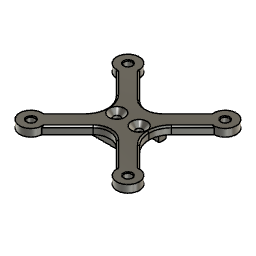
load_cell_contraption (Autodesk Fusion 360 archive; units mm, degrees)
design "Canon Weight Adapter"
Autodesk Fusion 360 part; units mm, degrees
sketch "Skizze1" plane through (0, 0, 0) normal (0, 0, 1) x (1, 0, 0)
  circle A0 centre (0, 0) radius 2.25
  line L0 (0, 0) -> (15, 0) construction
  circle A1 centre (15, 0) radius 2.25
  line L1 (-6.5, 6.5) -> (21.5, 6.5)
  line L2 (21.5, 0.0034) -> (21.5, -0.0034)
  line L3 (21.5, -6.5) -> (-6.5, -6.5)
  line L4 (-6.5, -0.0034) -> (-6.5, 0.0034)
  line L5 (21.5, -11.5) -> (-6.5, -11.5)
  line L6 (-6.5, 11.5) -> (21.5, 11.5)
  line L7 (-6.5, 6.5) -> (-6.5, 11.5)
  line L8 (-6.5, -6.5) -> (-6.5, -11.5)
  line L9 (21.5, 6.5) -> (21.5, 11.5)
  line L10 (21.5, -6.5) -> (21.5, -11.5)
  circle A2 centre (-25.006, 32.4943) radius 7.5
  circle A3 centre (-25.006, 32.4943) radius 2.5
  line L11 (-25.006, 32.4943) -> (7.5, 0) construction
  circle A4 centre (7.5, 0) radius 5.5 construction
  circle A5 centre (-25.006, 32.4943) radius 5.5 construction
  line L12 (-21.1176, 36.3841) -> (-0.2768, 15.5508)
  line L13 (-28.8944, 28.6045) -> (-10.8953, 10.6119)
  line L14 (-6.5, 0) -> (21.5, 0) construction
  line L15 (7.5, 11.5) -> (7.5, -11.5) construction
  circle A6 centre (40.006, 32.4943) radius 7.5
  circle A7 centre (40.006, 32.4943) radius 2.5
  line L16 (36.1176, 36.3841) -> (15.2768, 15.5508)
  line L17 (43.8944, 28.6045) -> (25.8953, 10.6119)
  circle A8 centre (40.006, -32.4943) radius 7.5
  line L18 (36.1176, -36.3841) -> (15.2768, -15.5508)
  line L19 (43.8944, -28.6045) -> (25.8953, -10.6119)
  circle A9 centre (40.006, -32.4943) radius 2.5
  line L20 (-21.1176, -36.3841) -> (-0.2768, -15.5508)
  line L21 (-28.8944, -28.6045) -> (-10.8953, -10.6119)
  circle A10 centre (-25.006, -32.4943) radius 7.5
  circle A11 centre (-25.006, -32.4943) radius 2.5
  arc A12 (-6.5, 0.0034) -> (-10.8953, 10.6119) centre (-21.5, 0.0034) ccw
  arc A13 (-10.8953, -10.6119) -> (-6.5, -0.0034) centre (-21.5, -0.0034) ccw
  arc A14 (25.8953, 10.6119) -> (21.5, 0.0034) centre (36.5, 0.0034) ccw
  arc A15 (21.5, -0.0034) -> (25.8953, -10.6119) centre (36.5, -0.0034) ccw
  arc A16 (-0.2768, 15.5508) -> (15.2768, 15.5508) centre (7.5, 23.3303) ccw
  arc A17 (15.2768, -15.5508) -> (-0.2768, -15.5508) centre (7.5, -23.3303) ccw
  dimension "d1" = 4.5
  dimension "d2" = 15
  dimension "d3" = 4.5
  dimension "d4" = 28
  dimension "d5" = 6.5
  dimension "d6" = 6.5
  dimension "d15" = 7.5
  dimension "d16" = 5
  dimension "d17" = 11
  dimension "d18" = 11
  dimension "d19" = 15
  dimension "d20" = 15
  dimension "d21" = 15
  dimension "d22" = 15
  dimension "d23" = 11
  dimension "d24" = 11
  constraint coincident A0.centre L0.start
  constraint horizontal L0
  constraint coincident L0.end A1.centre
  constraint horizontal L1
  constraint vertical L2
  constraint horizontal L3
  constraint vertical L4
  constraint perpendicular L6 L7
  constraint perpendicular L5 L8
  constraint perpendicular L6 L9
  constraint perpendicular L5 L10
  constraint concentric A2 A3
  constraint coincident A2.centre A3.centre
  constraint midpoint L0 L11.end
  constraint coincident L11.end A4.centre
  constraint concentric A3 A5
  constraint coincident A5 L12.start
  constraint tangent A4 L12
  constraint tangent A5 L12
  constraint coincident A5 L13.start
  constraint tangent A4 L13
  constraint tangent A5 L13
  constraint midpoint L6 L15.start
  constraint midpoint L5 L15.end
  constraint symmetric A2 L15 A6
  constraint symmetric A3 L15 A7
  constraint symmetric L12.start L15 L16.start
  constraint symmetric L13.start L15 L17.start
  constraint symmetric L0 A2 A10
  constraint symmetric L0 A3 A11
  constraint symmetric L0 L12.start L20.start
  constraint symmetric L0 L13.start L21.start
  constraint symmetric L0 A6 A8
  constraint symmetric L0 A7 A9
  constraint symmetric L0 L16.start L18.start
  constraint symmetric L0 L17.start L19.start
  constraint coincident L4 L14.start
  constraint coincident L1.start L4
  constraint tangent L13 A12
  constraint tangent L4 A12
  constraint coincident L3.end L4
  constraint tangent L21 A13
  constraint tangent L4 A13
  constraint coincident L2 L14.end
  constraint coincident L1.end L2
  constraint tangent L17 A14
  constraint tangent L2 A14
  constraint coincident L3.start L2
  constraint tangent L19 A15
  constraint tangent L2 A15
  constraint tangent L12 A16
  constraint tangent L16 A16
  constraint tangent L20 A17
  constraint tangent L18 A17
  measures "d1" diameter of A0
  measures "d2" distance of A0.centre L0.end
  measures "d3" diameter of A1
  measures "d4" distance of L1.start L1.end
  measures "d5" distance of A0.centre L1
  measures "d6" distance of A0.centre L4
  measures "d15" radius of A2
  measures "d16" diameter of A3
  measures "d17" diameter of A4
  measures "d18" diameter of A5
  measures "d19" radius of A12
  measures "d20" radius of A13
  measures "d21" radius of A14
  measures "d22" radius of A15
  measures "d23" radius of A16
  measures "d24" radius of A17
extrude "Extrusion1" add sketch "Skizze1" against normal blind 5 contours L1 L6 L7 L9 | L3 L5 L8 L10 makes body 1 at (12.1667, 9.8333, 0) makes body 2 at (12.1667, -11.5, -1.6667)
extrude "Extrusion2" add sketch "Skizze1" along normal blind 5 contours L1 L6 L7 L9 | L2 L4 A2 L12 L13 A6 L16 L17 A8 L18 L19 L20 L21 A10 A12 A13 A14 A15 A16 A17 | L3 L5 L8 L10 bodies 1 2
chamfer "Fase1" distance 3 angle 45 2 edges at (-2.0977, 0.8136, 5) (12.9023, 0.8136, 5) on bodies 1
extrude "Extrusion3" add sketch "Skizze1" along normal blind 5 contours A6 | A8 | A2 | A10 bodies 1
chamfer "Fase2" distance 1 angle 45 20 edges at (23.8941, 24.165, 5) (7.5, 12.3303, 5) (-8.8941, 24.165, 5) (33.0917, 17.8058, 5) (33.0917, -17.8058, 5) (22.6423, -5.7449, 5) (21.5, 0, 5) (22.6423, 5.7449, 5) (45.3103, 37.7967, 5) (23.8941, -24.165, 5) (-8.8941, -24.165, 5) (7.5, -12.3303, 5) (45.3103, -37.7967, 5) (-30.3103, -37.7967, 5) (-18.0917, -17.8058, 5) (-18.0917, 17.8058, 5) (-7.6423, 5.7449, 5) (-6.5, 0, 5) (-7.6423, -5.7449, 5) (-30.3103, 37.7967, 5) on bodies 1
extrude "Extrusion4" add sketch "Skizze1" along normal blind 5 contours A6 | A8 | A2 | A10 bodies 1
chamfer "Fase3" distance 0.5 angle 45 4 edges at (37.6752, -31.5903, 5) (-27.3368, -31.5903, 5) (-27.3368, 33.3984, 5) (37.6752, 33.3984, 5) on bodies 1
chamfer "Fase4" distance 0.5 angle 45 4 edges at (7.5, 6.5, -5) (7.5, -6.5, -5) (7.5, -11.5, -5) (7.5, 11.5, -5) on bodies 1
equation "d4 = 15 mm + 13 mm"

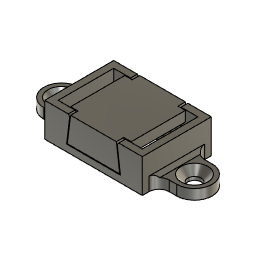
design "HX711 Cover"
Autodesk Fusion 360 part; units mm, degrees
sketch "Skizze1" plane through (0, 0, 0) normal (0, 0, 1) x (1, 0, 0)
  line L0 (0, 0) -> (25, 0)
  line L1 (25, 0) -> (25, 16.5)
  line L2 (25, 16.5) -> (0, 16.5)
  line L3 (0, 16.5) -> (0, 0)
  line L4 (3.5, 16.5) -> (3.5, 0)
  line L5 (21.5, 16.5) -> (21.5, 0)
  line L6 (-2, -2) -> (27, -2)
  line L7 (27, -2) -> (27, 18.5)
  line L8 (27, 18.5) -> (-2, 18.5)
  line L9 (-2, 18.5) -> (-2, -2)
  line L10 (5.5, 18.5) -> (5.5, -2)
  line L11 (19.5, 18.5) -> (19.5, -2)
  line L12 (12.5, -2) -> (12.5, 18.5) construction
  line L13 (12.5, 8.25) -> (27, 8.25) construction
  line L14 (27, 8.25) -> (32.25, 8.25) construction
  circle A0 centre (32.25, 8.25) radius 5.25
  circle A1 centre (32.25, 8.25) radius 3.25
  line L15 (32.25, 3) -> (27, 3)
  line L16 (32.25, 13.5) -> (27, 13.5)
  line L17 (-2, 8.25) -> (-7.25, 8.25) construction
  circle A2 centre (-7.25, 8.25) radius 3.25
  circle A3 centre (-7.25, 8.25) radius 5.25
  line L18 (-7.25, 3) -> (-2, 3)
  line L19 (-7.25, 13.5) -> (-2, 13.5)
  circle A4 centre (32.25, 8.25) radius 2
  circle A5 centre (-7.25, 8.25) radius 2
  line L20 (23, 14.5) -> (2, 14.5)
  line L21 (2, 14.5) -> (2, 2)
  line L22 (2, 2) -> (23, 2)
  line L23 (23, 2) -> (23, 14.5)
  dimension "d1" = 25
  dimension "d2" = 16.5
  dimension "d3" = 3.5
  dimension "d4" = 3.5
  dimension "d5" = 2
  dimension "d8" = 2
  dimension "d9" = 2
  dimension "d36" = 5.25
  dimension "d37" = 6.5
  dimension "d38" = 4
  dimension "d39" = 4
  dimension "d48" = -2
  constraint horizontal L0
  constraint vertical L1
  constraint horizontal L2
  constraint vertical L3
  constraint coincident L0.start L3.end
  constraint coincident L2 L4.start
  constraint coincident L0 L4.end
  constraint perpendicular L0 L4
  constraint coincident L2 L5.start
  constraint coincident L0 L5.end
  constraint perpendicular L0 L5
  constraint coincident L8 L10.start
  constraint coincident L6 L10.end
  constraint perpendicular L6 L10
  constraint coincident L8 L11.start
  constraint coincident L6 L11.end
  constraint perpendicular L6 L11
  constraint midpoint L6 L12.start
  constraint midpoint L8 L12.end
  constraint midpoint L12 L13.start
  constraint midpoint L7 L13.end
  constraint perpendicular L7 L14
  constraint coincident L14.end A0.centre
  constraint coincident L13.end A0
  constraint coincident A0 L15.start
  constraint coincident L7 L15.end
  constraint tangent A0 L15
  constraint perpendicular L7 L15
  constraint coincident A0 L16.start
  constraint coincident L7 L16.end
  constraint tangent A0 L16
  constraint perpendicular L7 L16
  constraint symmetric L12 L13.end L17.start
  constraint symmetric L12 L14.end L17.end
  constraint symmetric L12 A0 A3
  constraint symmetric L12 A1 A2
  constraint symmetric L12 L15.start L18.start
  constraint symmetric L12 L15.end L18.end
  constraint symmetric L12 L16.start L19.start
  constraint symmetric L12 L16.end L19.end
  constraint concentric A1 A4
  constraint concentric A2 A5
  measures "d1" distance of L0.start L0.end
  measures "d2" distance of L0.start L2.end
  measures "d3" distance of L3 L4
  measures "d4" distance of L1 L5
  measures "d8" distance of L4 L10
  measures "d9" distance of L5 L11
  measures "d36" distance of L13.end L14.end
  measures "d37" diameter of A1
  measures "d38" diameter of A4
  measures "d39" diameter of A5
extrude "Extrusion1" add sketch "Skizze1" against normal blind 2 contours L0 L2 L3 L4 L20 L21 L22 | L0 L2 L3 L6 L8 L9 L10 | L0 L4 L10 L22 | L0 L10 L11 L22 | L0 L6 L10 L11 | L4 L20 L21 L22 | L4 L10 L20 L22 | L2 L4 L10 L20 | L0 L5 L11 L22 | L0 L1 L2 L6 L7 L8 L11 | L10 L11 L20 L22 | L2 L8 L10 L11 | L2 L10 L11 L20 | L0 L1 L2 L5 L20 L22 L23 | L5 L11 L20 L22 | L2 L5 L11 L20 | L5 L20 L22 L23 makes body 1
extrude "Extrusion2" add sketch "Skizze1" along normal blind 6 contours L0 L2 L3 L6 L8 L9 L10 | L0 L1 L2 L6 L7 L8 L11 bodies 1
move_body "Verschieben1" bodies 1 to x (1, 0, 0) y (0, 1, 0) z (0, 0, 1) at (0, 0, -6)
extrude "Extrusion3" add sketch "Skizze1" along normal blind 2 contours L0 L2 L3 L6 L8 L9 L10 | L0 L1 L2 L6 L7 L8 L11 bodies 1
move_body "Verschieben2" bodies 1 to x (1, 0, 0) y (0, 1, 0) z (0, 0, 1) at (0, 0, -2)
extrude "Extrusion4" add sketch "Skizze1" against normal blind 2 separate body contours L0 L4 L10 L22 | L0 L10 L11 L22 | L0 L6 L10 L11 | L4 L10 L20 L22 | L2 L4 L10 L20 | L0 L5 L11 L22 | L10 L11 L20 L22 | L2 L8 L10 L11 | L2 L10 L11 L20 | L5 L11 L20 L22 | L2 L5 L11 L20 makes body 2
extrude "Extrusion5" add sketch "Skizze1" against normal blind 8 contours L0 L6 L10 L11 | L2 L8 L10 L11 bodies 2
sketch "Skizze2" plane through (0, 18.5, 0) normal (0, 1, 0) x (-1, 0, 0)
  line L0 (-27, 0) -> (-27, -10)
  line L1 (-27, -10) -> (2, -10)
  line L2 (2, -10) -> (2, 0)
  line L3 (2, 0) -> (-5.5, 0)
  line L4 (-5.5, 0) -> (-5.5, -8)
  line L5 (-5.5, -8) -> (-19.5, -8)
  line L6 (-19.5, -8) -> (-19.5, 0)
  line L7 (-19.5, 0) -> (-27, 0)
  line L8 (-19.5, 0) -> (-20.5, -8)
  line L9 (-20.5, -8) -> (-19.5, -8)
  line L10 (-5.5, -8) -> (-4.5, -8)
  line L11 (-4.5, -8) -> (-5.5, 0)
  line L12 (-19.5, -8) -> (-5.5, -8)
  line L13 (-19.3015, -0.0248) -> (-20.2734, -7.8)
  line L14 (-20.2734, -7.8) -> (-19.5, -7.8)
  line L15 (-19.5, -7.8) -> (-5.5, -7.8)
  line L16 (-5.5, -7.8) -> (-4.7266, -7.8)
  line L17 (-4.7266, -7.8) -> (-5.6985, -0.0248)
  line L18 (-19.5, 0) -> (-5.5, 0)
  line L19 (-5.6985, -0.0248) -> (-5.7016, 0)
  line L20 (-19.3015, -0.0248) -> (-19.2984, 0)
  dimension "d18" = -0.2
  constraint coincident L6.end L7.start
  constraint coincident L5.end L6.start
  constraint coincident L4.end L5.start
  constraint perpendicular L4 L10
  constraint coincident L3.end L4.start
  constraint parallel L17 L19
  constraint parallel L13 L20
  constraint coincident L18 L20.end
  constraint coincident L18 L19.end
extrude "Extrusion6" cut sketch "Skizze2" against normal blind 25 contours L6 L8 L9 L13 L14 | L6 L13 L14 | L4 L10 L11 L16 L17 | L4 L16 L17 bodies 1
extrude "Extrusion7" cut sketch "Skizze2" against normal blind 34 contours L4 L5 L6 L12 L15 bodies 2
extrude "Extrusion8" add sketch "Skizze2" against normal blind 20.5 contours L6 L13 L14 | L4 L16 L17 bodies 2
extrude "Extrusion9" cut sketch "Skizze2" against normal blind 18.5 contours L6 L13 L14 | L4 L16 L17 bodies 2
extrude "Extrusion10" add sketch "Skizze2" against normal blind 2 separate body contours L6 L13 L14 | L4 L16 L17 makes body 3 at (4.9844, 17.8333, -5.7375) makes body 4 at (19.7578, 17.8333, -3.675)
extrude "Extrusion11" cut sketch "Skizze2" against normal blind 21.5 contours L6 L13 L18 L20 | L4 L17 L18 L19 bodies 2
extrude "Extrusion12" add sketch "Skizze2" against normal blind 18.5 separate body contours L6 L13 L18 L20 | L4 L17 L18 L19 makes body 5 at (19.4328, 12.3333, -1.075) makes body 6 at (5.5672, 12.3333, -1.075)
extrude "Extrusion13" cut sketch "Skizze2" against normal blind 2 contours L6 L13 L18 L20 | L4 L17 L18 L19 bodies 5 6
combine "Kombinieren1" operation add target body 3 tool bodies 2 5 6 4
chamfer "Fase1" distance 0.5 angle 45 4 edges at (5.5, 17.5, 0) (19.5, 17.5, 0) (19.5, -1, 0) (5.5, -1, 0) on bodies 1
extrude "Extrusion14" add sketch "Skizze1" against normal blind 10 contours L9 A3 L18 | L7 A0 L15 | L9 A3 L19 | A3 | L7 A0 L16 | A0 | A1 | A2 bodies 1
extrude "Extrusion15" cut sketch "Skizze1" against normal blind 7 contours L9 A3 L18 | L7 A0 L15 | L9 A3 L19 | A3 | L7 A0 L16 | A0 | A1 | A2 bodies 1
chamfer "Fase2" distance 2 angle 45 2 edges at (30.3853, 7.5268, -7) (-9.1147, 7.5268, -7) on bodies 1
fillet "Abrundung1" radius 3 4 edges at (27, 13.5, -8.5) (-2, 13.5, -8.5) (-2, 3, -8.5) (27, 3, -8.5) on bodies 1
chamfer "Fase3" distance 1 angle 45 2 edges at (27, 8.25, -7) (-2, 8.25, -7) on bodies 1
extrude "Extrusion16" cut sketch "Skizze1" against normal blind 17 contours L4 L20 L21 L22 | L4 L10 L20 L22 | L10 L11 L20 L22 | L5 L11 L20 L22 | L5 L20 L22 L23 bodies 1
extrude "Extrusion17" cut 2 faces at (20.8333, 16.5, -1.2042) (4.1667, 16.5, -1.2042) along direction (0, -1, 0) blind 0.2 on bodies 3 bodies 3
extrude "Extrusion18" cut 2 faces at (20.8333, 0, -1.2042) (4.1667, 0, -1.2042) along direction (0, 1, 0) blind 0.2 on bodies 3 bodies 3
extrude "Extrusion19" add 1 faces at (2, 10.3333, -8.6667) along direction (1, 0, 0) blind 1 on bodies 1 bodies 1
extrude "Extrusion20" add 1 faces at (3, 10.3333, -8.6667) along direction (1, 0, 0) blind 1 on bodies 1 bodies 1
extrude "Extrusion21" add 1 faces at (23, 6.1667, -8.6667) along direction (-1, 0, 0) blind 2 on bodies 1 bodies 1
sketch "Skizze3" plane through (25, 0, 0) normal (-1, 0, 0) x (0, -1, 0)
  line L0 (-16.5, -8) -> (0, -8)
  line L1 (0, -8) -> (0, 0)
  line L2 (0, 0) -> (-16.5, 0)
  line L3 (-16.5, 0) -> (-16.5, -8)
extrude "Extrusion22" add 2 faces at (4.801, 5.5667, -2) (20.199, 10.9333, -2) along direction (0, 0, -1) blind 1 on bodies 3 bodies 3
extrude "Extrusion23" add 1 faces at (19.5484, 5.5667, -2.6667) along direction (-1, 0, 0) blind 14.5 on bodies 3 bodies 3
extrude "Extrusion24" add 2 faces at (10.1667, 16.3667, -2) (10.1667, 0.0667, -2) along direction (0, 0, -1) blind 1 on bodies 3 bodies 3
